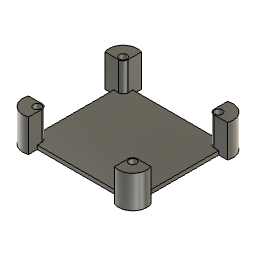
orangeBoxUp (Autodesk Fusion 360 design; units mm, degrees)
Autodesk Fusion 360 part; units mm, degrees
sketch "Sketch1" plane through (0, 0, 0) normal (0, 0, 1) x (1, 0, 0)
  line L0 (0, 0) -> (60, 0)
  line L1 (60, 0) -> (60, 60)
  line L2 (60, 60) -> (0, 60)
  line L3 (0, 60) -> (0, 0)
  line L4 (2, 2) -> (58, 2)
  line L5 (58, 2) -> (58, 58)
  line L6 (58, 58) -> (2, 58)
  line L7 (2, 58) -> (2, 2)
  dimension "d1" = 60
  dimension "d2" = 60
  dimension "d3" = 56
  dimension "d4" = 56
  constraint horizontal L0
  constraint vertical L1
  constraint horizontal L2
  constraint vertical L3
  constraint coincident L0.start L3.end
  constraint horizontal L4
  constraint vertical L5
  constraint horizontal L6
  constraint vertical L7
  measures "d1" distance of L0.start L0.end
  measures "d2" distance of L0.start L2.end
  measures "d3" distance of L4.start L4.end
  measures "d4" distance of L4.start L6.end
sketch "Sketch2" plane through (0, 0, 2) normal (0, 0, 1) x (-1, 0, 0)
  line L0 (-2, -2) -> (-4.5, -2)
  line L1 (-4.5, -2) -> (-4.5, -5)
  line L2 (-4.5, -5) -> (-2, -5)
  line L3 (-2, -5) -> (-2, -2)
  line L4 (-2, -58) -> (-4.5, -58)
  line L5 (-4.5, -58) -> (-4.5, -55)
  line L6 (-4.5, -55) -> (-2, -55)
  line L7 (-2, -55) -> (-2, -58)
  line L8 (-58, -58) -> (-49.5, -58)
  line L9 (-49.5, -58) -> (-49.5, -55)
  line L10 (-49.5, -55) -> (-58, -55)
  line L11 (-58, -55) -> (-58, -58)
  line L12 (-58, -2) -> (-49.5, -2)
  line L13 (-49.5, -2) -> (-49.5, -5)
  line L14 (-49.5, -5) -> (-58, -5)
  line L15 (-58, -5) -> (-58, -2)
  circle A0 centre (-4.5, -55) radius 1
  circle A1 centre (-49.5, -55) radius 1
  circle A2 centre (-4.5, -5) radius 1
  circle A3 centre (-49.5, -5) radius 1
  line L16 (-2, -58) -> (-2, -2)
  line L17 (-2, -2) -> (-58, -2)
  line L18 (-58, -2) -> (-58, -58)
  line L19 (-58, -58) -> (-2, -58)
  dimension "d9" = 2.5
  dimension "d10" = 3
  dimension "d11" = 2.5
  dimension "d12" = 3
  dimension "d13" = 8.5
  dimension "d14" = 3
  dimension "d15" = 8.5
  dimension "d16" = 3
  dimension "d17" = 2
  dimension "d18" = 2
  dimension "d19" = 2
  dimension "d20" = 2
  constraint horizontal L0
  constraint vertical L1
  constraint horizontal L2
  constraint vertical L3
  constraint horizontal L4
  constraint vertical L5
  constraint horizontal L6
  constraint vertical L7
  constraint horizontal L8
  constraint vertical L9
  constraint horizontal L10
  constraint vertical L11
  constraint horizontal L12
  constraint vertical L13
  constraint horizontal L14
  constraint vertical L15
  constraint coincident L5.end L6.start
  constraint coincident L9.end L10.start
  constraint coincident L1.end L2.start
  constraint coincident L13.end L14.start
  measures "d9" distance of L0.start L0.end
  measures "d10" distance of L0.start L2.end
  measures "d11" distance of L4.start L4.end
  measures "d12" distance of L4.start L6.end
  measures "d13" distance of L8.start L8.end
  measures "d14" distance of L8.start L10.end
  measures "d15" distance of L12.start L12.end
  measures "d16" distance of L12.start L14.end
  measures "d17" diameter of A0
  measures "d18" diameter of A1
  measures "d19" diameter of A2
  measures "d20" diameter of A3
sketch "Sketch3" plane through (0, 0, 0) normal (0, 0, 1) x (1, 0, 0)
  circle A0 centre (0, 45) radius 2
  circle A1 centre (50, 45) radius 2
  circle A2 centre (50, 0) radius 2
  circle A3 centre (0, 0) radius 2
  line L0 (0, -2.5) -> (50, -2.5)
  line L1 (52.5, 0) -> (52.5, 45)
  line L2 (-2.5, 0.0027) -> (-2.5, 45)
  line L3 (0.0001, 47.5) -> (50, 47.5)
  circle A4 centre (0, 45) radius 7.5
  circle A5 centre (0, 0) radius 7.5
  circle A6 centre (50, 45) radius 7.5
  circle A7 centre (50, 0) radius 7.5
  line L4 (0, 42.5) -> (-7.0711, 42.5)
  line L5 (2.5, 45) -> (2.5, 52.0711)
  line L6 (47.5, 45) -> (47.5, 52.0711)
  line L7 (50, 42.5) -> (57.0711, 42.5)
  line L8 (50, 2.5) -> (57.0711, 2.5)
  line L9 (47.5, 0) -> (47.5, -7.0711)
  line L10 (0, 2.5) -> (-7.0711, 2.5)
  line L11 (2.5, 0) -> (2.5, -7.0711)
  arc A8 (0, 42.5) -> (2.5, 45) centre (0, 45) ccw
  arc A9 (0.0001, 47.5) -> (-2.5, 45) centre (0, 45) ccw
  line L12 (0, 45) -> (0, 43)
  line L13 (2, 45) -> (0, 45)
  arc A10 (47.5, 45) -> (50, 42.5) centre (50, 45) ccw
  arc A11 (52.5, 45) -> (50, 47.5) centre (50, 45) ccw
  line L14 (50, 43) -> (50, 45)
  line L15 (50, 45) -> (48, 45)
  line L16 (47.5, 45) -> (2.5, 45)
  arc A12 (50, 2.5) -> (47.5, 0) centre (50, 0) ccw
  arc A13 (50, -2.5) -> (52.5, 0) centre (50, 0) ccw
  line L17 (48, 0) -> (50, 0)
  line L18 (50, 0) -> (50, 2)
  line L19 (50, 2.5) -> (50, 42.5)
  arc A14 (-2.5, 0.0027) -> (0, -2.5) centre (0, 0) ccw
  arc A15 (2.5, 0) -> (0, 2.5) centre (0, 0) ccw
  line L20 (0, 0) -> (2, 0)
  line L21 (2.5, 0) -> (47.5, 0)
  line L22 (0, 42.5) -> (0, 2.5)
  line L23 (0, 2) -> (0, 0)
  dimension "d23" = 50
  dimension "d24" = 45
  dimension "d25" = 4
  dimension "d26" = 4
  dimension "d27" = 4
  dimension "d28" = 4
  dimension "d29" = 5
  dimension "d30" = 5
  dimension "d31" = 5
  dimension "d32" = 5
  dimension "d37" = 15
  dimension "d38" = 15
  dimension "d39" = 15
  dimension "d40" = 15
  constraint horizontal L20
  constraint vertical L18
  constraint horizontal L15
  constraint vertical L12
  constraint coincident A3.centre A5.centre
  constraint coincident A0.centre A4.centre
  constraint coincident A1.centre A6.centre
  constraint coincident A2.centre A7.centre
  constraint concentric A0 A8
  constraint concentric A1 A10
  constraint concentric A2 A12
  constraint coincident L0.end A12
  constraint tangent L0 A12
  constraint perpendicular L0 L12
  constraint coincident L1.end A10
  constraint tangent L1 A10
  constraint perpendicular L0 L1
  constraint tangent L2 A8
  constraint coincident L3.start A8
  constraint tangent L3 A10
  constraint concentric A0 A4
  constraint concentric A1 A6
  constraint concentric A7 A12
  constraint coincident L4.start L12
  constraint coincident A4 L4.end
  constraint tangent L4 A8
  constraint coincident A4 L5.end
  constraint tangent L5 A8
  constraint coincident L6.start L15
  constraint coincident A6 L6.end
  constraint tangent L6 A10
  constraint perpendicular L3 L6
  constraint coincident A6 L7.end
  constraint tangent L7 A10
  constraint coincident L8.start L18
  constraint coincident A7 L8.end
  constraint tangent L8 A12
  constraint coincident A7 L9.end
  constraint tangent L9 A12
  constraint coincident L10.start L12
  constraint coincident A5 L10.end
  constraint tangent L10 A14
  constraint coincident L11.start A14
  constraint coincident L11.start L20
  constraint coincident A5 L11.end
  constraint tangent L11 A14
  constraint concentric A8 A9
  constraint coincident A0 L12.end
  constraint collinear L12 L22
  constraint coincident A0 L13.start
  constraint collinear L13 L15
  constraint concentric A10 A11
  constraint coincident A1 L14.start
  constraint collinear L14 L18
  constraint coincident A1 L15.end
  constraint collinear L15 L16
  constraint concentric A12 A13
  constraint coincident A2 L17.start
  constraint collinear L17 L20
  constraint coincident A2 L18.end
  constraint collinear L18 L19
  constraint concentric A14 A15
  constraint coincident A3 L20.end
  constraint collinear L20 L21
  constraint coincident A3 L23.start
  constraint collinear L22 L23
  measures "d23" distance of A3.centre A2.centre
  measures "d24" distance of A3.centre A0.centre
  measures "d25" diameter of A0
  measures "d26" diameter of A1
  measures "d27" diameter of A2
  measures "d28" diameter of A3
  measures "d29" diameter of A14
  measures "d30" diameter of A8
  measures "d31" diameter of A10
  measures "d32" diameter of A12
  measures "d37" diameter of A4
  measures "d38" diameter of A5
  measures "d39" diameter of A6
  measures "d40" diameter of A7
extrude "Extrude6" add sketch "Sketch3" along normal blind 7 contours L0 L2 A5 L10 L11 A14 | L0 L1 A7 L8 L9 A13 | L2 L3 A4 L4 L5 A9 | L1 L3 A6 L6 L7 A11 makes body 1 at (48.1731, 52.2741, 2.3333) makes body 2 at (48.8622, -7.4132, 4.6667) makes body 3 at (-7.4132, 43.8622, 2.3333) makes body 4 at (2.1658, -7.1805, 4.6667)
extrude "Extrude7" add sketch "Sketch3" along normal blind 2 separate body contours L0 A5 L11 L21 | L0 A5 A7 L21 | A5 A15 L21 L22 | L2 A5 L10 L22 | L0 A7 L9 L21 | A4 A5 A6 A7 L16 L19 L21 L22 | L2 A4 A5 L22 | A7 A12 L19 L21 | L2 A4 L4 L22 | L1 A6 A7 L19 | L1 A7 L8 L19 | A4 A8 L16 L22 | L1 A6 L7 L19 | A6 A10 L16 L19 | L3 A4 L5 L16 | L3 A4 A6 L16 | L3 A6 L6 L16 makes body 5
extrude "Extrude8" add sketch "Sketch3" along normal blind 6 contours L0 L2 L10 L11 A14 A15 | L0 L1 L8 L9 A12 A13 | L2 L3 L4 L5 A8 A9 | L1 L3 L6 L7 A10 A11 bodies 1 2 3 4 5
sketch "Sketch4" plane through (0, 0, 7) normal (0, 0, 1) x (-1, 0, 0)
  line L0 (-2.5, -47.5) -> (-2.5, -52.0711)
  arc A0 (-2.5, -52.0711) -> (7.0711, -42.5) centre (0, -45) ccw
  line L1 (7.0711, -42.5) -> (2.5, -42.5)
  line L2 (2.5, -42.5) -> (2.5, -45)
  arc A1 (-0.0001, -47.5) -> (2.5, -45) centre (0, -45) ccw
  line L3 (-0.0001, -47.5) -> (-2.5, -47.5)
  line L4 (3.0524, -42.5) -> (-2.4476, -42.5)
  line L5 (-2.4476, -42.5) -> (-2.4476, -48)
  line L6 (-2.4476, -48) -> (3.0524, -48)
  line L7 (3.0524, -48) -> (3.0524, -42.5)
  line L8 (-53.0435, -42.4424) -> (-47.5435, -42.4424)
  line L9 (-47.5435, -42.4424) -> (-47.5435, -47.9424)
  line L10 (-47.5435, -47.9424) -> (-53.0435, -47.9424)
  line L11 (-53.0435, -47.9424) -> (-53.0435, -42.4424)
  line L12 (-47, 3) -> (-53, 3)
  line L13 (-53, 3) -> (-53, -3)
  line L14 (-53, -3) -> (-47, -3)
  line L15 (-47, -3) -> (-47, 3)
  line L16 (-3, 3) -> (3, 3)
  line L17 (3, 3) -> (3, -3)
  line L18 (3, -3) -> (-3, -3)
  line L19 (-3, -3) -> (-3, 3)
  dimension "d47" = 5.5
  dimension "d48" = 5.5
  dimension "d49" = 5.5
  dimension "d50" = 5.5
  constraint horizontal L4
  constraint vertical L5
  constraint horizontal L6
  constraint vertical L7
  constraint coincident L1 L4.start
  constraint horizontal L8
  constraint vertical L9
  constraint horizontal L10
  constraint vertical L11
  constraint horizontal L12
  constraint vertical L13
  constraint horizontal L14
  constraint vertical L15
  constraint horizontal L16
  constraint vertical L17
  constraint horizontal L18
  constraint vertical L19
  measures "d47" distance of L4.start L4.end
  measures "d48" distance of L4.start L6.end
  measures "d49" distance of L8.start L8.end
  measures "d50" distance of L8.start L10.end
extrude "Extrude9" cut sketch "Sketch4" against normal blind 1 contours L1 L2 A1 L3 L4 L5 L6 L7 | L8 L9 L10 L11 | L12 L13 L14 L15 | L16 L17 L18 L19 bodies 1
extrude "Extrude10" cut 4 faces at (52.6956, 45.1475, 6) (-2.7016, 45.1667, 6) (-0.1168, -2.6648, 6) (50.2165, -2.6648, 6) along direction (0, 0, -1) blind 1 on bodies 1 bodies 1
extrude "Extrude11" cut 4 faces at (50.4007, 49.4532, 7) (50.3718, -4.4916, 7) (-4.4916, -0.3718, 7) (-0.4067, 49.4916, 7) along direction (0, 0, -1) blind 1 on bodies 1 bodies 1
extrude "Extrude12" add 4 faces at (-2.7016, 45.1667, 5) (52.6956, 45.1475, 5) (50.2165, -2.6648, 5) (-0.1168, -2.6648, 5) along direction (0, 0, 1) blind 12 on bodies 1 bodies 1
sketch "Sketch5" plane through (0, 0, 17) normal (0, 0, 1) x (-1, 0, 0)
  circle A0 centre (-50, -45) radius 2
  line L0 (-47.5435, -47.5) -> (-47.5, -47.5)
  line L1 (-47.5, -47.5) -> (-47.5, -45)
  arc A1 (-47.5, -45) -> (-50, -42.5) centre (-50, -45) ccw
  line L2 (-50, -42.5) -> (-53.0435, -42.5)
  line L3 (-53.0435, -42.5) -> (-53.0435, -47.9424)
  line L4 (-53.0435, -47.9424) -> (-47.5435, -47.9424)
  line L5 (-47.5435, -47.9424) -> (-47.5435, -47.5)
  circle A2 centre (-50, -45) radius 3
  circle A3 centre (0, -45) radius 3
  circle A4 centre (0, 0) radius 3
  circle A5 centre (-50, 0) radius 3
  line L6 (-47, 3) -> (-53, 3)
  line L7 (-53, 3) -> (-53, -3)
  line L8 (-53, -3) -> (-47, -3)
  line L9 (-47, -3) -> (-47, 3)
  line L10 (-47.0435, -44.4912) -> (-47.0435, -45.5088)
  line L11 (-49.5553, -47.9669) -> (-50.4447, -47.9669)
  line L12 (-3, -42) -> (3, -42)
  line L13 (3, -42) -> (3, -48)
  line L14 (3, -48) -> (-3, -48)
  line L15 (-3, -48) -> (-3, -42)
  line L16 (-3, -3) -> (3, -3)
  line L17 (3, -3) -> (3, 3)
  line L18 (3, 3) -> (-3, 3)
  line L19 (-3, 3) -> (-3, -3)
  line L20 (-53.0435, -47.9669) -> (-53.0435, -47.9424)
  line L21 (-53.0435, -42.5) -> (-53.0435, -41.9669)
  line L22 (-47, -42) -> (-53.4773, -42)
  line L23 (-53.4773, -42) -> (-53.4773, -48.6117)
  line L24 (-53.4773, -48.6117) -> (-47, -48.6117)
  line L25 (-47, -48.6117) -> (-47, -42)
  dimension "d59" = 6
  dimension "d60" = 6
  dimension "d61" = 6
  dimension "d62" = 6
  dimension "d64" = 6
  constraint concentric A0 A2
  constraint coincident A4.centre origin
  constraint horizontal L6
  constraint vertical L7
  constraint horizontal L8
  constraint vertical L9
  constraint vertical L10
  constraint horizontal L11
  constraint vertical L20
  constraint horizontal L12
  constraint vertical L13
  constraint horizontal L14
  constraint vertical L15
  constraint horizontal L16
  constraint vertical L17
  constraint horizontal L18
  constraint vertical L19
  constraint coincident A2 L10.start
  constraint coincident A2 L10.end
  constraint coincident A2 L11.start
  constraint coincident A2 L11.end
  constraint collinear L20 L21
  constraint horizontal L22
  constraint vertical L23
  constraint horizontal L24
  constraint vertical L25
  measures "d59" diameter of A2
  measures "d60" diameter of A3
  measures "d61" diameter of A4
  measures "d62" diameter of A5
  measures "d64" distance of L21.end L20.start
extrude "Extrude13" cut sketch "Sketch5" against normal blind 11 contours L0 L1 L4 L5 A2 | L0 L1 L3 L4 L5 A2 L21 L22 L23 L24 L25 | L2 L3 L4 A2 | A3 L13 L14 | A3 L12 L13 | A3 L14 L15 | A4 L16 L17 | A4 L17 L18 | A4 L18 L19 | A5 L6 L9 | A5 L6 L7 | A5 L7 L8 bodies 1
delete_face "DeleteFace1" 1 faces at (-3.0524, 46.1667, 9.6667) on bodies 1
sketch "Sketch6" plane through (0, 0, 2) normal (0, 0, 1) x (-1, 0, 0)
  line L0 (-2.5, 2.5) -> (-47.5, 2.5)
  line L1 (-47.5, 2.5) -> (-47.5, 0)
  arc A0 (-50, -2.5) -> (-47.5, 0) centre (-50, 0) ccw
  line L2 (-50, -2.5) -> (-52.5, -2.5)
  line L3 (-52.5, -2.5) -> (-52.5, -42.5)
  line L4 (-52.5, -42.5) -> (-50, -42.5)
  arc A1 (-47.5, -45) -> (-50, -42.5) centre (-50, -45) ccw
  line L5 (-47.5, -45) -> (-47.5, -47.5)
  line L6 (-47.5, -47.5) -> (-2.5, -47.5)
  line L7 (-2.5, -47.5) -> (-2.5, -45)
  arc A2 (0, -42.5) -> (-2.5, -45) centre (0, -45) ccw
  line L8 (0, -42.5) -> (2.5, -42.5)
  line L9 (2.5, -42.5) -> (2.5, -2.5)
  line L10 (2.5, -2.5) -> (0, -2.5)
  arc A3 (-2.5, 0) -> (0, -2.5) centre (0, 0) ccw
  line L11 (-2.5, 0) -> (-2.5, 2.5)
  line L12 (2.5, -42.5) -> (-3.5, -42.5)
  line L13 (-3.5, -42.5) -> (-3.5, -40.5)
  line L14 (-3.5, -40.5) -> (2.5, -40.5)
  line L15 (2.5, -40.5) -> (2.5, -42.5)
  line L16 (2.5, -40.5) -> (-3.5, -40.5)
  line L17 (-3.5, -40.5) -> (-3.5, -4.5)
  line L18 (-3.5, -4.5) -> (2.5, -4.5)
  line L19 (2.5, -4.5) -> (2.5, -40.5)
  line L20 (-52.5, -42.5) -> (-46.5, -42.5)
  line L21 (-46.5, -42.5) -> (-46.5, -40.5)
  line L22 (-46.5, -40.5) -> (-52.5, -40.5)
  line L23 (-52.5, -40.5) -> (-52.5, -42.5)
  line L24 (-46.5, -40.5) -> (-52.5, -40.5)
  line L25 (-52.5, -40.5) -> (-52.5, -4.5)
  line L26 (-52.5, -4.5) -> (-46.5, -4.5)
  line L27 (-46.5, -4.5) -> (-46.5, -40.5)
  dimension "d67" = 6
  dimension "d68" = 2
  dimension "d69" = 6
  dimension "d70" = 36
  dimension "d71" = 6
  dimension "d72" = 2
  dimension "d73" = 6
  dimension "d74" = 36
  constraint horizontal L12
  constraint vertical L13
  constraint horizontal L14
  constraint vertical L15
  constraint coincident L8.end L9.start
  constraint horizontal L16
  constraint vertical L17
  constraint horizontal L18
  constraint vertical L19
  constraint horizontal L20
  constraint vertical L21
  constraint horizontal L22
  constraint vertical L23
  constraint coincident L3.end L4.start
  constraint horizontal L24
  constraint vertical L25
  constraint horizontal L26
  constraint vertical L27
  measures "d67" distance of L8.end L12.end
  measures "d68" distance of L8.end L14.end
  measures "d69" distance of L14.end L13.end
  measures "d70" distance of L14.end L18.end
  measures "d71" distance of L3.end L20.end
  measures "d72" distance of L3.end L22.end
  measures "d73" distance of L21.end L22.end
  measures "d74" distance of L21.end L26.end
extrude "Extrude14" cut sketch "Sketch6" against normal blind 2 contours L9 L14 L16 L17 L18 L19 | L3 L22 L24 L25 L26 L27 bodies 1
extrude "Extrude15" add sketch "Sketch6" against normal blind 2 contours L9 L14 L16 L17 L18 L19 | L3 L22 L24 L25 L26 L27 bodies 1
extrude "Extrude16" add 4 faces at (49.8538, 49.4573, 6) (48.4271, -5.7771, 6) (1.5729, -5.7771, 6) (-5.7771, 43.4271, 6) along direction (0, 0, 1) blind 11 on bodies 1 bodies 1
